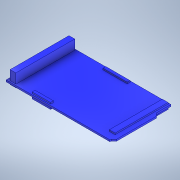
# Autodesk Inventor part: Adaptateur écran_carte
Saved by Autodesk Inventor 2020 (Build 240168000, 168)
## iProperties
Created: 2020-01-01
Part Number: Adaptateur écran_carte
Material: Argent
Document SubType Name: Modeling
Designer: Manuel Enzo
Density: 10.49 g/cm^3
Appearance: Bleu - Peinture murale - Brillant
Author: Manuel Enzo
Autodesk Inventor part; units mm, degrees
ref_plane "YZ Plane" through (0, 0, 0) normal (1, 0, 0) x (0, 1, 0)
ref_plane "XZ Plane" through (0, 0, 0) normal (0, 1, 0) x (-1, 0, 0)
ref_plane "XY Plane" through (0, 0, 0) normal (0, 0, 1) x (1, 0, 0)
sketch "Esquisse1" plane through (0, 0, 0) normal (0, 1, 0) x (-1, 0, 0)
  line L0 (0, 0) -> (90, 0)
  line L1 (90, 0) -> (90, -53)
  line L2 (90, -53) -> (0, -53)
  line L3 (0, -53) -> (0, 0)
  line L4 (0, -3.5) -> (-2.5, -3.5)
  line L5 (-2.5, -3.5) -> (-2.5, -38)
  line L6 (-2.5, -38) -> (0, -38)
  line L7 (0, -38) -> (0, -3.5)
  line L8 (-2.5, -38) -> (0, -40.5)
  line L9 (-2.5, -3.5) -> (0, -1)
  line L10 (87.5, -1) -> (82.5, -1)
  line L11 (82.5, -1) -> (82.5, -52)
  line L12 (82.5, -52) -> (87.5, -52)
  line L13 (87.5, -52) -> (87.5, -1)
  dimension "d0" = 90
  dimension "d1" = 53
  dimension "d2" = 15
  dimension "d3" = 3.5
  dimension "d4" = 2.5
  dimension "d5" = 45
  dimension "d6" = 45
  dimension "d7" = 2.5
  dimension "d8" = 1
  dimension "d9" = 1
  dimension "d10" = 5
  constraints: 28 end point, 6 parallel, 4 perpendicular, 3 horizontal, 3 point on line
  measures "d0" distance between parallel lines of L3 L1
  measures "d1" distance between parallel lines of L0 L2
  measures "d2" distance between parallel lines of L2 L6
  measures "d3" distance between parallel lines of L0 L4
  measures "d4" distance between parallel lines of L3 L5
  measures "d5" angle of L4 L9
  measures "d6" angle of L8 L6
  measures "d7" distance between parallel lines of L1 L13
  measures "d8" distance between parallel lines of L12 L2
  measures "d9" distance between parallel lines of L0 L10
  measures "d10" distance between parallel lines of L11 L13
extrude "Extrusion1" add sketch "Esquisse1" along normal blind 1.5 contours L0 L1 L2 L3 | L3 L4 L9 | L3 L6 L5 L4 | L3 L8 L6 | L13 L12 L11 L10
extrude "Extrusion2" add sketch "Esquisse1" along normal blind 10 contours L13 L12 L11 L10
sketch "Esquisse2" plane through (0, 0, 0) normal (0, -1, 0) x (1, 0, 0)
  line L0 (-1.5, -52) -> (-6.5, -52)
  line L1 (-6.5, -52) -> (-6.5, -6)
  line L2 (-6.5, -6) -> (-1.5, -6)
  line L3 (-1.5, -6) -> (-1.5, -52)
  line L4 (0, -53) -> (-90, -53) projected
  line L5 (0, -40.5) -> (0, -53) projected
  line L6 (-90, 0) -> (0, 0) projected
  line L7 (-34.5, -49.5) -> (-55.5, -49.5)
  line L8 (-55.5, -49.5) -> (-55.5, -52)
  line L9 (-55.5, -52) -> (-34.5, -52)
  line L10 (-34.5, -52) -> (-34.5, -49.5)
  line L11 (-52.5, -1) -> (-68.5, -1)
  line L12 (-68.5, -1) -> (-68.5, -3.5)
  line L13 (-68.5, -3.5) -> (-52.5, -3.5)
  line L14 (-52.5, -3.5) -> (-52.5, -1)
  dimension "d15" = 1
  dimension "d16" = 1.5
  dimension "d17" = 5
  dimension "d18" = 46
  dimension "d19" = 6
  dimension "d20" = 34.5
  dimension "d21" = 21
  dimension "d22" = 2.5
  dimension "d23" = 1
  dimension "d24" = 52.5
  dimension "d25" = 16
  dimension "d26" = 1
  dimension "d27" = 2.5
  constraints: 24 end point, 6 parallel, 3 horizontal, 3 perpendicular
  measures "d15" distance between parallel lines of L4 L0
  measures "d16" distance between parallel lines of L5 L3
  measures "d17" distance between parallel lines of L1 L3
  measures "d18" distance between parallel lines of L2 L0
  measures "d19" distance between parallel lines of L6 L2
  measures "d20" distance between parallel lines of L5 L10
  measures "d21" distance between parallel lines of L8 L10
  measures "d22" distance between parallel lines of L9 L7
  measures "d23" distance between parallel lines of L4 L9
  measures "d24" distance between parallel lines of L14 L5
  measures "d25" distance between parallel lines of L12 L14
  measures "d26" distance between parallel lines of L6 L11
  measures "d27" distance between parallel lines of L11 L13
extrude "Extrusion3" add sketch "Esquisse2" along normal blind 2.5
extrude "Extrusion4" add sketch "Esquisse1" against normal blind 1.25 contours L13 L12 L11 L10
extrude "Extrusion5" add sketch "Esquisse2" against normal blind 2.75 contours L10 L9 L8 L7
extrude "Extrusion6" add sketch "Esquisse2" against normal blind 2.75 contours L0 L1 L2 L3 | L14 L13 L12 L11
